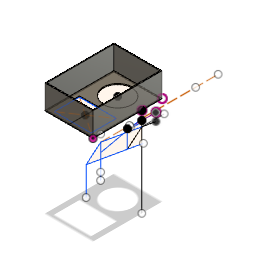
YI (Autodesk Fusion 360 design; units mm, degrees)
Autodesk Fusion 360 part; units mm, degrees
note: some values were not read from the file. Set by a fixed rule: which sketch regions a step uses.
sketch "Sketch1" plane through (0, 0, 0) normal (0, 1, 0) x (1, 0, 0)
  line L0 (0, 0) -> (-44, 0)
  line L1 (-44, 0) -> (-44, 63)
  line L2 (-44, 63) -> (0, 63)
  line L3 (0, 63) -> (0, 0)
  line L4 (-22, 0) -> (-22, 15)
  line L5 (-44, 0) -> (-22, 0)
  line L6 (-22, 0) -> (-22, 63)
  line L7 (-22, 63) -> (-22, 44.5)
  circle A0 centre (-22, 44.5) radius 13
  line L8 (-44, 63) -> (-22, 63)
  line L9 (-5.2012, 3.5077) -> (-38.7988, 3.5077)
  line L10 (-38.7988, 3.5077) -> (-38.7988, 26.4923)
  line L11 (-38.7988, 26.4923) -> (-5.2012, 26.4923)
  line L12 (-5.2012, 26.4923) -> (-5.2012, 3.5077)
  line L13 (-5.2012, 3.5077) -> (-38.7988, 26.4923) construction
  line L14 (-38.7988, 3.5077) -> (-5.2012, 26.4923) construction
  line L15 (-43, 62) -> (-1, 62)
  line L16 (-1, 62) -> (-1, 1)
  line L17 (-1, 1) -> (-43, 1)
  line L18 (-43, 1) -> (-43, 62)
  dimension "d1" = 44
  dimension "d2" = 63
  dimension "d5" = 15
  dimension "d7" = 18.5
  dimension "d8" = 26
  dimension "d9" = 21
  dimension "d13" = 21.5
  dimension "d14" = 1
  measures "d5" distance of L0.start
  measures "d8" diameter of A0
extrude "Extrude3" add sketch "Sketch1" along normal blind 22 contours L0 L2 L3 L4 L6 L7 L15 L16 L17 | L0 L1 L2 L4 L5 L6 L7 L8 L15 L17 L18 makes body 1
extrude "Extrude2" add sketch "Sketch1" along normal blind 1 separate body contours L0 L2 L3 L4 L6 L7 L15 L16 L17 | L0 L1 L2 L4 L5 L6 L7 L8 L15 L17 L18 | L4 L6 L7 A0 L9 L10 L11 L15 L17 L18 | L4 L6 L7 A0 L9 L11 L12 L15 L16 L17 makes body 2
combine "Combine1" operation add target body 1 tool bodies 2
extrude "Extrude5" add sketch "Sketch1" along normal blind 21 separate body contours L4 L6 L7 A0 L9 L10 L11 L15 L17 L18 | L4 L6 L7 A0 L9 L11 L12 L15 L16 L17 | L4 L6 L9 L10 L11 | L4 L6 L9 L11 L12 | L6 L7 A0 | L6 L7 A0 makes body 3
move_body "Move1" bodies 3 to x (1, 0, 0) y (0, 1, 0) z (0, 0, 1) at (0, 1, 0)
extrude "Extrude6" add sketch "Sketch1" along normal blind -8 and the other way blind -1 separate body contours L6 L7 A0 | L6 L7 A0 makes body 4
combine "Combine2" operation add target body 4 tool bodies 3
sketch "Sketch3" plane through (0, 0, 0) normal (1, 0, 0) x (0, 0, -1)
  line L0 (44.5, -8) -> (44.5, -95.3333)
  line L1 (44.5, -8) -> (44.5007, 25.9882)
  line L2 (44.5, -8) -> (44.5, -13)
  line L3 (44.5, -8) -> (44.5, -13)
  line L4 (44.5, -8) -> (44.5, -13)
  line L5 (44.5, -5.7455) -> (28.5885, -9.273)
  line L6 (44.5, -5.7455) -> (93.193, -5.7455) construction
  line L7 (44.5, -5.7455) -> (101.0974, -5.7455) construction
  line L8 (44.5, -9.273) -> (25, -9.273)
  line L9 (28.5885, -9.273) -> (28.5885, -28.9115)
  line L10 (28.5885, -28.9115) -> (23.5129, -33.9871)
  line L11 (44.5, -13) -> (73.6492, -13) construction
  line L12 (44.5, -13) -> (28.5885, -28.9115)
  line L13 (28.5885, -28.9115) -> (-8.934, -28.9115)
  line L14 (44.5, -13) -> (28.5885, -13)
  line L15 (44.5, -13) -> (7, -12.9775)
  line L16 (7, -12.9775) -> (30.0264, -12.9775) construction
  line L17 (7, -12.9775) -> (-8.934, -28.9115)
  line L18 (-8.934, -28.9115) -> (-8.934, -33.9115)
  line L19 (6.9775, -13) -> (6.9775, -33.9115)
  line L20 (28.5885, -13) -> (6.9775, -13)
  line L21 (-8.934, -28.9115) -> (-8.934, -33.9115)
  line L22 (-8.934, -33.9115) -> (6.9775, -33.9115)
  line L23 (6.9775, -33.9115) -> (44.5, -42.23)
  line L24 (6.9775, -33.9115) -> (31.1364, -33.9115) construction
  line L25 (-8.934, -33.9115) -> (-89.4653, -51.7648)
  line L26 (-8.934, -33.9115) -> (73.5526, -33.9115) construction
  dimension "d31" = 5
  dimension "d36" = 45
  dimension "d37" = 77.5
  dimension "d38" = 37.5
  dimension "d40" = 12.5
  dimension "d41" = 167.5
  measures "d36" angle of L0 L10
  measures "d37" angle of L0 L5
  measures "d40" angle of L23 L24
  measures "d41" angle of L25 L26
sketch "Sketch4" plane through (0, 0, 0) normal (1, 0, 0) x (0, 0, -1)
  line L0 (63, 0) -> (44.5, 0)
  line L1 (44.5, 0) -> (44.5, -81.2522)
  line L2 (31.5, -8) -> (57.5, -8)
  line L3 (44.5, -8) -> (57, -8)
  line L4 (44.5, -6.4048) -> (93.5414, -6.4048) construction
  line L5 (44.5, -8) -> (44.5, -13)
  line L6 (44.5, -8) -> (31.5, -8)
  line L7 (31.5, -8) -> (34.5, -8)
  line L8 (44.5, -6.3277) -> (113.977, -6.3277) construction
  line L9 (44.5, -9.2652) -> (31.25, -9.2652)
  line L10 (31.25, -9.2652) -> (31.25, -24.1181)
  line L11 (44.5, -13) -> (31.25, -24.1181)
  line L12 (44.5, -13) -> (64.8642, -13) construction
  line L13 (44.5, -13) -> (7, -6.3877)
  line L14 (57.3025, -15.2574) -> (44.5, -13)
  line L15 (45.8772, -26.6972) -> (-6.25, -17.5058)
  line L16 (44.5, 0) -> (7, 0)
  line L17 (7, -6.3877) -> (7, -30)
  line L18 (7, -6.3877) -> (-6.25, -17.5058)
  line L19 (7, -6.3877) -> (33.2311, -6.3877) construction
  line L20 (44.5, -6.3277) -> (7, -14.6413)
  line L21 (-6.25, -17.5058) -> (-6.25, -43.4537)
  line L22 (7, -14.6413) -> (7, -36.5614)
  line L23 (7, -6.3877) -> (7, -14.6413)
  dimension "d44" = 5
  dimension "d46" = 3
  dimension "d47" = 167.5
  dimension "d49" = 50
  dimension "d50" = 37.5
  dimension "d51" = 140
  measures "d47" angle of L8 L20
  measures "d49" angle of L1 L11
  measures "d50" distance of origin
  measures "d51" angle of L18 L19
hidden bodies 4
